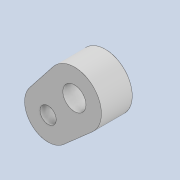
# Autodesk Inventor part: IRLedMount
Saved by Autodesk Inventor 2020 (Build 240168000, 168)
## iProperties
Created: 2021-07-27
Part Number: IRLedMount
Material: Generic
Document SubType Name: Modeling
Designer: Val
Density: 1 g/cm^3
Appearance: Default
Author: Val
Autodesk Inventor part; units mm, degrees
ref_plane "YZ Plane" through (0, 0, 0) normal (1, 0, 0) x (0, 1, 0)
ref_plane "XZ Plane" through (0, 0, 0) normal (0, 1, 0) x (-1, 0, 0)
sketch "Base" plane through (0, 0, 0) normal (0, 0, 1) x (1, 0, 0)
  circle A0 centre (-17.02, -17.02) radius 1.05 projected
  arc A1 (-12.5579, -14.4893) -> (-14.6643, -12.3531) centre (-13.6111, -13.4212) ccw construction
  line L0 (-13.6111, -13.4212) -> (-17.02, -17.02) construction
  circle A2 centre (-13.6111, -13.4212) radius 1.5
  circle A3 centre (-13.6111, -13.4212) radius 3.5
  circle A4 centre (-17.02, -17.02) radius 3.05
  line L1 (-11.2991, -16.0489) -> (-15.0053, -19.3098)
  line L2 (-16.3601, -11.2549) -> (-19.4156, -15.1322)
  point P0 (0, 0)
  point P1 (-15.3155, -15.2206)
  dimension "d3" = 2
  dimension "d4" = 2
  constraints: 8 end point, 4 point on circle, 4 tangent, 3 coincident, 2 centre point, 1 midpoint, 3 other
  measures "d3" radial gap between concentric circles of A3 A1
  measures "d4" radial gap between concentric circles of A4 A0
extrude "BaseFeature" add sketch "Base" along normal blind 7
ref_plane "RisePlane" through (0, 0, 3) normal (0, 0, 1) x (1, 0, 0)
sketch "RiseProfile" plane through (0, 0, 0) normal (0, 0, -1) x (-1, 0, 0)
  arc A0 (15.0053, -19.3098) -> (19.4156, -15.1322) centre (17.02, -17.02) ccw projected
  line L0 (16.3601, -11.2549) -> (19.4156, -15.1322) projected
  circle A1 centre (17.02, -17.02) radius 3.05
  line L1 (15.0053, -19.3098) -> (11.2991, -16.0489) projected
  arc A2 (16.3601, -11.2549) -> (11.2991, -16.0489) centre (13.6111, -13.4212) ccw projected
  point P0 (0, 0)
  point P1 (15.0053, -19.3098)
  constraints: 1 coincident, 3 other
extrude "RiseFeature" cut sketch "RiseProfile" against normal up to surface (3 mm away) contours L1 A2 L0 A1
body "Solid1"
